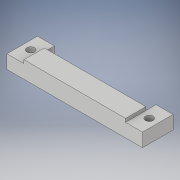
# Autodesk Inventor part: ABI_KastenSchnitt
Saved by Autodesk Inventor 2018.3 (Build 223284000, 284)
## iProperties
Created: 2019-11-22
Part Number: ABI_KastenSchnitt
Material: Generisch
Document SubType Name: Modeling
Designer: maascl
Density: 1 g/cm^3
Appearance: Vorgabe
Author: maascl
Autodesk Inventor part; units mm, degrees
ref_plane "YZ Plane" through (0, 0, 0) normal (1, 0, 0) x (0, 1, 0)
ref_plane "XZ Plane" through (0, 0, 0) normal (0, 1, 0) x (-1, 0, 0)
ref_plane "XY Plane" through (0, 0, 0) normal (0, 0, 1) x (1, 0, 0)
sketch "Skizze1" plane through (0, 0, 0) normal (0, 0, 1) x (1, 0, 0)
  line L0 (-40, 9) -> (40, 9)
  line L1 (40, 9) -> (40, -9)
  line L2 (40, -9) -> (-40, -9)
  line L3 (-40, -9) -> (-40, 9)
  line L4 (-40, 9) -> (40, -9) construction
  line L5 (40, 9) -> (-40, -9) construction
  point P0 (0, 0)
  dimension "Breite" = 80
  dimension "d1" = 18
  constraints: 12 end point, 2 midpoint, 2 parallel, 1 horizontal, 1 perpendicular
  measures "Breite" distance between parallel lines of L1 L3
  measures "d1" distance between parallel lines of L0 L2
extrude "Extrusion1" add sketch "Skizze1" along normal blind 10
sketch "Skizze2" plane through (0, 0, 10) normal (0, 0, 1) x (1, 0, 0)
  line L0 (-56, 0) -> (56, 0) projected
  line L1 (0, -12.6) -> (0, 12.6) projected
  line L2 (40, 9) -> (-40, 9) projected
  line L3 (-40, 9) -> (-40, -9) projected
  line L4 (-40, -9) -> (40, -9) projected
  line L5 (40, -9) -> (40, 9) projected
  line L6 (30, 3) -> (-30, 3)
  line L7 (-30, 3) -> (-30, 9)
  line L8 (-30, 9) -> (30, 9)
  line L9 (30, 9) -> (30, 3)
  line L10 (30, 3) -> (-30, 9) construction
  line L11 (-30, 3) -> (30, 9) construction
  point P0 (0, 0)
  point P1 (0, 6)
  dimension "d4" = 60
  dimension "d5" = 6
  constraints: 12 end point, 2 midpoint, 2 parallel, 2 point on line, 1 horizontal, 1 perpendicular
  measures "d4" distance of L6.start L6.end
  measures "d5" distance of L6.end L7.end
extrude "Extrusion2" cut sketch "Skizze2" against normal through all contours L6 L7 L2 L1 | L1 L2 L9 L6
sketch "Skizze3" plane through (0, 0, 10) normal (0, 0, 1) x (1, 0, 0)
  line L0 (-30, 9) -> (-40, 9) projected
  line L1 (-30, 9) -> (-40, 9)
  line L2 (-40, 9) -> (-40, -9)
  line L3 (-40, -9) -> (-30, -9)
  line L4 (-30, -9) -> (-30, 9)
  point P0 (0, 0)
  constraints: 8 end point, 2 parallel, 1 horizontal, 1 perpendicular
extrude "Extrusion3" cut sketch "Skizze3" against normal blind 2
sketch "Skizze4" plane through (0, 0, 10) normal (0, 0, 1) x (1, 0, 0)
  line L0 (40, 9) -> (30, 9)
  line L1 (30, 9) -> (30, -9)
  line L2 (30, -9) -> (40, -9)
  line L3 (40, -9) -> (40, 9)
  point P0 (0, 0)
  constraints: 8 end point, 2 parallel, 1 horizontal, 1 perpendicular
extrude "Extrusion4" cut sketch "Skizze4" against normal blind 2
sketch "Skizze5" plane through (0, 0, 0) normal (0, 0, -1) x (-1, 0, 0)
  line L0 (0, -12.6) -> (0, 12.6) projected
  line L1 (-30, 9) -> (-40, 9) projected
  point P0 (0, 0)
  point P1 (-35, 0)
  point P2 (35, 0)
  dimension "d12" = 9
  constraints: 1 symmetric about line
  measures "d12" distance from line of L1 point (-35, 0)
hole "Bohrung1" at (35, 0, 0) at (-35, 0, 0) direction (0, 0, 1) diameter 4.5 end through all counterbore diameter 8 counterbore depth 4.6
